test (Autodesk Fusion 360 design; units mm, degrees)
Autodesk Fusion 360 part; units mm, degrees
sketch "Sketch1" plane through (0, 0, 0) normal (0, 0, 1) x (1, 0, 0)
  line L0 (36.4, -60.9) -> (-36.4, -60.9)
  line L1 (-36.4, -60.9) -> (-36.4, 60.9)
  line L2 (-36.4, 60.9) -> (36.4, 60.9)
  line L3 (36.4, 60.9) -> (36.4, -60.9)
  line L4 (36.4, -60.9) -> (-36.4, 60.9) construction
  line L5 (-36.4, -60.9) -> (36.4, 60.9) construction
  line L6 (26.4, -50.9) -> (-26.4, -50.9) construction
  line L7 (-26.4, -50.9) -> (-26.4, 50.9) construction
  line L8 (-26.4, 50.9) -> (26.4, 50.9) construction
  line L9 (26.4, 50.9) -> (26.4, -50.9) construction
  line L10 (26.4, -50.9) -> (-26.4, 50.9) construction
  line L11 (-26.4, -50.9) -> (26.4, 50.9) construction
  circle A0 centre (-26.4, 50.9) radius 2.1
  circle A1 centre (26.4, 50.9) radius 2.1
  circle A2 centre (26.4, -50.9) radius 2.1
  circle A3 centre (-26.4, -50.9) radius 2.1
  dimension "d1" = 121.8
  dimension "d2" = 101.8
  dimension "d3" = 52.8
  dimension "d4" = 10
  dimension "d5" = 4.2
  dimension "d6" = 4.2
  dimension "d7" = 4.2
  dimension "d8" = 4.2
  constraint horizontal L0
  constraint perpendicular L0 L1
  constraint parallel L0 L2
  constraint parallel L1 L3
  constraint coincident L4 origin
  constraint coincident L5 origin
  constraint horizontal L6
  constraint perpendicular L6 L7
  constraint parallel L6 L8
  constraint parallel L7 L9
  constraint coincident L10 origin
  constraint coincident L11 origin
  constraint coincident L7.end L8.start
  constraint coincident L8.end L9.start
  constraint coincident L6.start L9.end
  constraint coincident L6.end L7.start
  measures "d1" distance of L0.end L1.end
  measures "d2" distance of L6.end L7.end
  measures "d3" distance of L7.end L8.end
  measures "d4" horizontal distance of L2.end L8.end
  measures "d5" diameter of A0
  measures "d6" diameter of A1
  measures "d7" diameter of A2
  measures "d8" diameter of A3
extrude "Extrude1" add sketch "Sketch1" along normal blind 4
equation "d2 = ( 50.9 * 2 ) * 1 mm"
